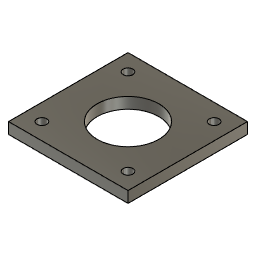
Tilt motor spacer (Autodesk Fusion 360 design; units mm, degrees)
Autodesk Fusion 360 part; units mm, degrees
sketch "Szkic1" plane through (0, 0, 0) normal (0, 0, 1) x (1, 0, 0)
  line L0 (0, 0) -> (43, 0)
  line L1 (43, 0) -> (43, 43)
  line L2 (43, 43) -> (0, 43)
  line L3 (0, 43) -> (0, 0)
  line L4 (37, 6) -> (6, 37) construction
  line L5 (6, 6) -> (37, 37) construction
  circle A0 centre (6, 37) radius 1.75
  circle A1 centre (37, 37) radius 1.75
  circle A2 centre (37, 6) radius 1.75
  circle A3 centre (6, 6) radius 1.75
  circle A4 centre (21.5, 21.5) radius 11.1
  point P0 (21.5, 21.5)
  dimension "d1" = 43
  dimension "d2" = 43
  dimension "d3" = 31
  dimension "d4" = 31
  dimension "d5" = 3.5
  dimension "d6" = 3.5
  dimension "d7" = 3.5
  dimension "d8" = 3.5
  dimension "d9" = 22.2
  constraint horizontal L0
  constraint vertical L1
  constraint horizontal L2
  constraint vertical L3
  constraint coincident L0.start L3.end
  constraint coincident L4 P0
  constraint coincident L5 P0
  constraint coincident L4.end A0.centre
  constraint coincident L5.end A1.centre
  constraint coincident L4.start A2.centre
  constraint coincident L5.start A3.centre
  constraint coincident P0 A4.centre
  measures "d1" distance of L0.start L0.end
  measures "d2" distance of L0.start L2.end
  measures "d3" distance of L4.end L5.end
  measures "d4" distance of L5.start L4.end
  measures "d5" diameter of A0
  measures "d6" diameter of A1
  measures "d7" diameter of A2
  measures "d8" diameter of A3
  measures "d9" diameter of A4
extrude "Wyciągnięcie proste1" add sketch "Szkic1" along normal blind 4
